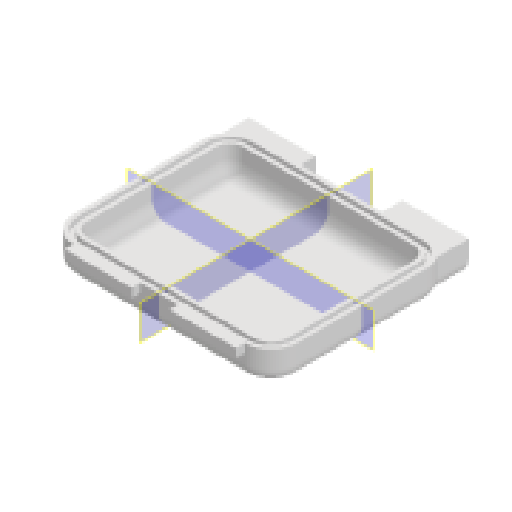
# Autodesk Inventor part: 00_OutdoorCase_Type2000_toplid
Saved by Autodesk Inventor 2024.1 (Build 281209000, 209)
## iProperties
Created: 2024-06-29
Part Number: 00_OutdoorCase_Type2000_toplid
Material: Generisch
Document SubType Name: Modeling
Designer: diederichbenedict
Density: 1 g/cm^3
Appearance: Vorgabe
Mass: 806.448 g
Surface Area: 1765.71 cm^2
Volume: 806.448 cm^3
Author: diederichbenedict
Autodesk Inventor part; units mm, degrees
ref_plane "YZ Plane" through (0, 0, 0) normal (1, 0, 0) x (0, 1, 0)
ref_plane "XZ Plane" through (0, 0, 0) normal (0, 1, 0) x (-1, 0, 0)
ref_plane "XY Plane" through (0, 0, 0) normal (0, 0, 1) x (1, 0, 0)
sketch "Skizze1" plane through (0, 0, 0) normal (0, 0, 1) x (1, 0, 0)
  line L0 (0, 0) -> (446.8518, 0) construction
  line L1 (446.8518, 0) -> (446.8519, -335.1389) construction
  line L2 (446.8519, -335.1389) -> (0, -335.1389) construction
  line L3 (0, -335.1389) -> (0, 0) construction
  line L4 (0, 0) -> (446.8519, 0)
  line L5 (446.8519, 0) -> (446.8519, -335.1389)
  line L6 (446.8519, -335.1389) -> (0, -335.1389)
  line L7 (0, -335.1389) -> (0, 0)
  line L8 (248.7149, -119.366) -> (248.7149, -159.1284)
  line L9 (149.5274, -83.4391) -> (352.5274, -83.4391)
  line L10 (367.5274, -98.4391) -> (367.5274, -246.4391)
  line L11 (352.5274, -261.4391) -> (149.5274, -261.4391)
  line L12 (134.5274, -246.4391) -> (134.5274, -98.4391)
  arc A0 (149.5274, -83.4391) -> (134.5274, -98.4391) centre (149.5274, -98.4391) ccw
  arc A1 (134.5274, -246.4391) -> (149.5274, -261.4391) centre (149.5274, -246.4391) ccw
  arc A2 (352.5274, -261.4391) -> (367.5274, -246.4391) centre (352.5274, -246.4391) ccw
  arc A3 (367.5274, -98.4391) -> (352.5274, -83.4391) centre (352.5274, -98.4391) ccw
  line L13 (119.5274, -98.4391) -> (119.5274, -246.4391)
  arc A4 (119.5274, -246.4391) -> (149.5274, -276.4391) centre (149.5274, -246.4391) ccw
  line L14 (149.5274, -276.4391) -> (352.5274, -276.4391)
  arc A5 (352.5274, -276.4391) -> (382.5274, -246.4391) centre (352.5274, -246.4391) ccw
  line L15 (382.5274, -246.4391) -> (382.5274, -98.4391)
  arc A6 (382.5274, -98.4391) -> (352.5274, -68.4391) centre (352.5274, -98.4391) ccw
  line L16 (352.5274, -68.4391) -> (149.5274, -68.4391)
  arc A7 (149.5274, -68.4391) -> (119.5274, -98.4391) centre (149.5274, -98.4391) ccw
  line L17 (200.5274, -51.4391) -> (124.5274, -51.4391)
  line L18 (124.5274, -51.4391) -> (124.5274, -81.8559)
  line L19 (124.5274, -81.8559) -> (200.5274, -81.8559)
  line L20 (200.5274, -81.8559) -> (200.5274, -51.4391)
  line L21 (301.5274, -45.4625) -> (377.5274, -45.4625)
  line L22 (377.5274, -45.4625) -> (377.5274, -81.8559)
  line L23 (377.5274, -81.8559) -> (301.5274, -81.8559)
  line L24 (301.5274, -81.8559) -> (301.5274, -45.4625)
  point P0 (367.5274, -261.4391)
  point P1 (367.5274, -83.4391)
  point P2 (134.5274, -261.4391)
  point P3 (200.5274, -68.4391)
  point P4 (301.5274, -68.4391)
  dimension "d10" = 233
  dimension "d11" = 178
  dimension "d13" = 15
  dimension "d14" = 15
  dimension "d24" = 5
  dimension "d25" = 17
  dimension "d26" = 76
  dimension "d27" = 5
  dimension "d28" = 76
  constraints: 42 end point, 18 point on circle, 10 parallel, 8 centre point, 8 tangent, 6 point on line, 5 perpendicular, 4 horizontal, 3 equal radius, 1 coincident, 9 other
  measures "d10" distance of point (367.527, -261.439) point (134.527, -261.439)
  measures "d11" distance of point (367.527, -83.439) point (367.527, -261.439)
  measures "d13" radius of A0
  measures "d14" distance between parallel lines of L12 L13
  measures "d24" distance between parallel lines of L18 L13
  measures "d25" distance between parallel lines of L16 L17
  measures "d26" distance between parallel lines of L20 L18
  measures "d27" distance between parallel lines of L22 L15
  measures "d28" distance between parallel lines of L22 L24
extrude "Extrusion1" add sketch "Skizze1" along normal blind 30 contours A7 L19 L20 L16 L24 L23 A6 L15 A5 L14 A4 L13 | L18 L17 L20 L16 A7 | A7 L16 L20 L19 | L24 L21 L22 A6 L16 | L16 A6 L23 L24
sketch "Skizze2" plane through (0, 0, 0) normal (0, 0, -1) x (-1, 0, 0)
  arc A0 (-149.5274, -276.4391) -> (-119.5274, -246.4391) centre (-149.5274, -246.4391) ccw projected
  line L0 (-119.5274, -98.4391) -> (-119.5274, -246.4391) projected
  arc A1 (-119.5274, -98.4391) -> (-124.5274, -81.8559) centre (-149.5274, -98.4391) ccw projected
  line L1 (-301.5274, -68.4391) -> (-200.5274, -68.4391) projected
  arc A2 (-377.5274, -81.8559) -> (-382.5274, -98.4391) centre (-352.5274, -98.4391) ccw projected
  line L2 (-382.5274, -246.4391) -> (-382.5274, -98.4391) projected
  arc A3 (-382.5274, -246.4391) -> (-352.5274, -276.4391) centre (-352.5274, -246.4391) ccw projected
  line L3 (-149.5274, -276.4391) -> (-352.5274, -276.4391) projected
  line L4 (-134.5274, -246.4391) -> (-134.5274, -98.4391) projected
  arc A4 (-149.5274, -261.4391) -> (-134.5274, -246.4391) centre (-149.5274, -246.4391) ccw projected
  line L5 (-352.5274, -261.4391) -> (-149.5274, -261.4391) projected
  arc A5 (-367.5274, -246.4391) -> (-352.5274, -261.4391) centre (-352.5274, -246.4391) ccw projected
  line L6 (-367.5274, -98.4391) -> (-367.5274, -246.4391) projected
  arc A6 (-352.5274, -83.4391) -> (-367.5274, -98.4391) centre (-352.5274, -98.4391) ccw projected
  line L7 (-149.5274, -83.4391) -> (-352.5274, -83.4391) projected
  arc A7 (-134.5274, -98.4391) -> (-149.5274, -83.4391) centre (-149.5274, -98.4391) ccw projected
  line L8 (-124.5274, -51.4391) -> (-124.5274, -81.8559) projected
  line L9 (-200.5274, -51.4391) -> (-124.5274, -51.4391) projected
  line L10 (-200.5274, -68.4391) -> (-200.5274, -51.4391) projected
  line L11 (-301.5274, -45.4625) -> (-301.5274, -68.4391) projected
  line L12 (-377.5274, -45.4625) -> (-301.5274, -45.4625) projected
  line L13 (-377.5274, -81.8559) -> (-377.5274, -45.4625) projected
  point P0 (0, 0)
extrude "Extrusion2" add sketch "Skizze2" along normal blind 6 contours L3 A3 L2 A2 L13 L12 L11 L1 L10 L9 L8 A1 L0 A0 | A4 L5 A5 L6 A6 L7 A7 L4
fillet "Rundung1" radius 15 20 edges at (381.2502, -89.7788, -6) (382.5274, -172.4391, -6) (373.7406, -267.6523, -6) (251.0274, -276.4391, -6) (128.3142, -267.6523, -6) (119.5274, -172.4391, -6) (120.8046, -89.7788, -6) (251.0274, -68.4391, -6) (363.134, -87.8325, 0) (367.5274, -172.4391, 0) (363.134, -257.0457, 0) (251.0274, -261.4391, 0) (138.9208, -257.0457, 0) (134.5274, -172.4391, 0) (138.9208, -87.8325, 0) (251.0274, -83.4391, 0) (200.5274, -59.9391, -6) (301.5274, -56.9508, -6) (124.5274, -66.6475, -6) (377.5274, -63.6592, -6)
sketch "Skizze3" plane through (0, 0, 30) normal (0, 0, 1) x (1, 0, 0)
  arc A0 (119.5274, -246.4391) -> (149.5274, -276.4391) centre (149.5274, -246.4391) ccw projected
  line L0 (149.5274, -276.4391) -> (352.5274, -276.4391) projected
  arc A1 (352.5274, -276.4391) -> (382.5274, -246.4391) centre (352.5274, -246.4391) ccw projected
  line L1 (382.5274, -246.4391) -> (382.5274, -98.4391) projected
  arc A2 (382.5274, -98.4391) -> (377.5274, -81.8559) centre (352.5274, -98.4391) ccw projected
  line L2 (301.5274, -68.4391) -> (200.5274, -68.4391) projected
  arc A3 (124.5274, -81.8559) -> (119.5274, -98.4391) centre (149.5274, -98.4391) ccw projected
  line L3 (119.5274, -98.4391) -> (119.5274, -246.4391) projected
  line L4 (134.5274, -246.4391) -> (134.5274, -98.4391) projected
  arc A4 (149.5274, -83.4391) -> (134.5274, -98.4391) centre (149.5274, -98.4391) ccw projected
  line L5 (149.5274, -83.4391) -> (352.5274, -83.4391) projected
  arc A5 (367.5274, -98.4391) -> (352.5274, -83.4391) centre (352.5274, -98.4391) ccw projected
  line L6 (367.5274, -98.4391) -> (367.5274, -246.4391) projected
  arc A6 (352.5274, -261.4391) -> (367.5274, -246.4391) centre (352.5274, -246.4391) ccw projected
  line L7 (352.5274, -261.4391) -> (149.5274, -261.4391) projected
  arc A7 (134.5274, -246.4391) -> (149.5274, -261.4391) centre (149.5274, -246.4391) ccw projected
  line L8 (149.5274, -73.4391) -> (352.5274, -73.4391)
  arc A8 (377.5274, -98.4391) -> (352.5274, -73.4391) centre (352.5274, -98.4391) ccw
  line L9 (377.5274, -98.4391) -> (377.5274, -246.4391)
  arc A9 (352.5274, -271.4391) -> (377.5274, -246.4391) centre (352.5274, -246.4391) ccw
  line L10 (352.5274, -271.4391) -> (149.5274, -271.4391)
  arc A10 (124.5274, -246.4391) -> (149.5274, -271.4391) centre (149.5274, -246.4391) ccw
  line L11 (124.5274, -246.4391) -> (124.5274, -98.4391)
  arc A11 (149.5274, -73.4391) -> (124.5274, -98.4391) centre (149.5274, -98.4391) ccw
  line L12 (352.5274, -78.4391) -> (149.5274, -78.4391)
  arc A12 (149.5274, -78.4391) -> (129.5274, -98.4391) centre (149.5274, -98.4391) ccw
  line L13 (129.5274, -98.4391) -> (129.5274, -246.4391)
  arc A13 (129.5274, -246.4391) -> (149.5274, -266.4391) centre (149.5274, -246.4391) ccw
  line L14 (149.5274, -266.4391) -> (352.5274, -266.4391)
  arc A14 (352.5274, -266.4391) -> (372.5274, -246.4391) centre (352.5274, -246.4391) ccw
  line L15 (372.5274, -246.4391) -> (372.5274, -98.4391)
  arc A15 (372.5274, -98.4391) -> (352.5274, -78.4391) centre (352.5274, -98.4391) ccw
  line L16 (377.5274, -81.8559) -> (377.5274, -45.4625) projected
  line L17 (377.5274, -45.4625) -> (301.5274, -45.4625) projected
  line L18 (301.5274, -45.4625) -> (301.5274, -68.4391) projected
  line L19 (200.5274, -68.4391) -> (200.5274, -51.4391) projected
  line L20 (200.5274, -51.4391) -> (124.5274, -51.4391) projected
  line L21 (124.5274, -51.4391) -> (124.5274, -81.8559) projected
  point P0 (0, 0)
  dimension "d20" = 5
  dimension "d21" = 5
  constraints: 16 end point, 16 point on circle, 8 centre point, 14 other
  measures "d20" distance between parallel lines of L2 L8
  measures "d21" distance between parallel lines of L5 L12
extrude "Extrusion3" cut sketch "Skizze3" against normal blind 6 contours L8 A8 L9 A9 L10 A10 L11 A11
sketch "Skizze4" plane through (0, 0, 30) normal (0, 0, 1) x (1, 0, 0)
  arc A0 (119.5274, -246.4391) -> (149.5274, -276.4391) centre (149.5274, -246.4391) ccw projected
  line L0 (149.5274, -276.4391) -> (352.5274, -276.4391) projected
  arc A1 (352.5274, -276.4391) -> (382.5274, -246.4391) centre (352.5274, -246.4391) ccw projected
  line L1 (382.5274, -246.4391) -> (382.5274, -98.4391) projected
  arc A2 (382.5274, -98.4391) -> (377.5274, -81.8559) centre (352.5274, -98.4391) ccw projected
  line L2 (377.5274, -81.8559) -> (377.5274, -45.4625) projected
  line L3 (377.5274, -45.4625) -> (301.5274, -45.4625) projected
  line L4 (301.5274, -45.4625) -> (301.5274, -68.4391) projected
  line L5 (301.5274, -68.4391) -> (200.5274, -68.4391) projected
  line L6 (200.5274, -68.4391) -> (200.5274, -51.4391) projected
  line L7 (200.5274, -51.4391) -> (124.5274, -51.4391) projected
  line L8 (124.5274, -51.4391) -> (124.5274, -81.8559) projected
  arc A3 (124.5274, -81.8559) -> (119.5274, -98.4391) centre (149.5274, -98.4391) ccw projected
  line L9 (119.5274, -98.4391) -> (119.5274, -246.4391) projected
  arc A4 (352.5274, -271.4391) -> (377.5274, -246.4391) centre (352.5274, -246.4391) ccw projected
  line L10 (352.5274, -271.4391) -> (149.5274, -271.4391) projected
  arc A5 (124.5274, -246.4391) -> (149.5274, -271.4391) centre (149.5274, -246.4391) ccw projected
  line L11 (124.5274, -246.4391) -> (124.5274, -98.4391) projected
  arc A6 (149.5274, -73.4391) -> (124.5274, -98.4391) centre (149.5274, -98.4391) ccw projected
  line L12 (149.5274, -73.4391) -> (352.5274, -73.4391) projected
  arc A7 (377.5274, -98.4391) -> (352.5274, -73.4391) centre (352.5274, -98.4391) ccw projected
  line L13 (377.5274, -98.4391) -> (377.5274, -246.4391) projected
  line L14 (149.5274, -276.4391) -> (225.5274, -276.4391)
  line L15 (225.5274, -276.4391) -> (225.5274, -286.4391)
  line L16 (225.5274, -286.4391) -> (149.5274, -286.4391)
  line L17 (149.5274, -286.4391) -> (149.5274, -276.4391)
  line L18 (352.5274, -276.4391) -> (276.5274, -276.4391)
  line L19 (276.5274, -276.4391) -> (276.5274, -286.4391)
  line L20 (276.5274, -286.4391) -> (352.5274, -286.4391)
  line L21 (352.5274, -286.4391) -> (352.5274, -276.4391)
  point P0 (0, 0)
  dimension "d30" = 76
  dimension "d31" = 10
  dimension "d32" = 76
  constraints: 16 end point, 4 parallel, 2 horizontal, 2 perpendicular, 1 point on line
  measures "d30" distance of L15.end L16.end
  measures "d31" distance of L14.end L15.end
  measures "d32" distance of L20.end L19.end
extrude "Extrusion4" add sketch "Skizze4" against normal blind 10 contours L0 L15 L16 L17 | L0 L21 L20 L19
ref_plane "Arbeitsebene1" through (251.0274, -246.4391, 30) normal (-1, 0, 0) x (0, 0, 1)
ref_plane "Arbeitsebene2" through (200.5274, -172.4391, 30) normal (0, 1, 0) x (1, 0, 0)
